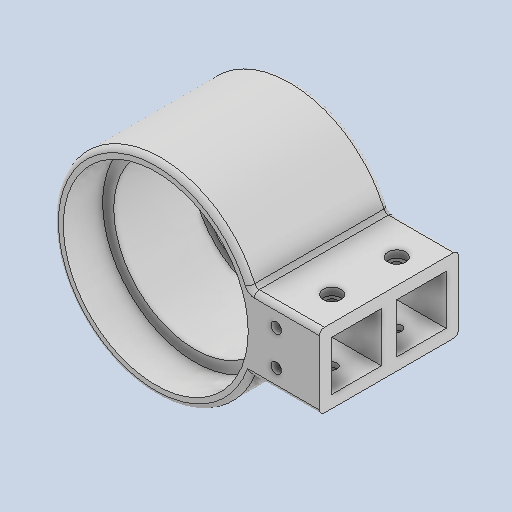
# Autodesk Inventor part: j2 arm part
Saved by Autodesk Inventor 2025 (Build 290162000, 162)
## iProperties
Created: 2025-07-06
Part Number: j2 arm part
Material: 一般
Document SubType Name: Modeling
Designer: gavin
Density: 1 g/cm^3
Appearance: 預設
Author: gavin
## iProperties of the stored document j2 arm part_3D 列印.ipt
Created: 2025-08-02
Part Number: j2 arm part_3D 列印
Material: 一般
Document SubType Name: Modeling
Designer: gavin
Density: 1 g/cm^3
Appearance: 預設
Author: gavin
Autodesk Inventor part; units mm, degrees
sketch "草圖1" plane through (0, 0, 0) normal (0, 0, 1) x (1, 0, 0)
  circle A0 centre (0, 0) radius 19.6
  circle A1 centre (0, 0) radius 41.575
  dimension "d0" = 39.2
  dimension "d1" = 83.15
  constraints: 2 centre point, 2 coincident
  measures "d0" diameter of A0
  measures "d1" diameter of A1
extrude "擠出1" add sketch "草圖1" along normal blind 5
sketch "草圖2" plane through (0, 0, 0) normal (0, 0, -1) x (-1, 0, 0)
  circle A0 centre (0, 0) radius 41.575 projected
extrude "擠出2" add sketch "草圖2" along normal blind 4
sketch "草圖4" plane through (0, 0, 5) normal (0, 0, 1) x (1, 0, 0)
  circle A0 centre (0, 0) radius 41.575 projected
  circle A1 centre (0, 0) radius 37.575
  dimension "d14" = 4
  constraints: 1 centre point
  measures "d14" radial gap between concentric circles of A0 A1
extrude "擠出4" add sketch "草圖4" along normal blind 47.5
sketch "草圖5" plane through (0, 0, 5) normal (0, 0, 1) x (1, 0, 0)
  circle A0 centre (0, 0) radius 37.575 projected
  circle A1 centre (0, 0) radius 33.075
  dimension "d17" = 4.5
  constraints: 1 centre point
  measures "d17" radial gap between concentric circles of A0 A1
extrude "擠出5" add sketch "草圖5" along normal blind 31.5
sketch "草圖6" plane through (0, 0, -4) normal (0, 0, -1) x (-1, 0, 0)
  line L0 (-66.575, 15.075) -> (-66.575, -15.075)
  line L1 (-66.575, 15.075) -> (-38.7456, 15.075)
  circle A0 centre (0, 0) radius 41.575 projected
  line L2 (-66.575, -15.075) -> (-38.7456, -15.075)
  point P0 (-41.575, 0)
  dimension "d20" = 30.15
  dimension "d22" = 15.075
  dimension "d25" = 25
  constraints: 6 end point, 3 point on circle, 2 horizontal, 1 vertical
  measures "d20" distance of L0.start L0.end
  measures "d22" distance from line of point (0, 0) L1
  measures "d25" distance from line of point (-41.575, 0) L0
extrude "擠出6" add sketch "草圖6" against normal up to surface (56.5 mm away) contours L1 A0 L2 L0
sketch "草圖7" plane through (66.575, -15.075, -4) normal (1, 0, 0) x (0, 0, -1)
  line L0 (-56.5, 30.15) -> (-56.5, 0) projected
  line L1 (0, 0) -> (-56.5, 0) projected
  line L2 (0, 30.15) -> (0, 0) projected
  line L3 (0, 30.15) -> (-56.5, 30.15) projected
  line L4 (-51.5, 5) -> (-31.35, 5)
  line L5 (-31.35, 5) -> (-31.35, 25.15)
  line L6 (-31.35, 25.15) -> (-51.5, 25.15)
  line L7 (-51.5, 25.15) -> (-51.5, 5)
  line L8 (-51.5, 5) -> (-31.35, 25.15) construction
  line L9 (-31.35, 5) -> (-51.5, 25.15) construction
  line L10 (-25.15, 5.0185) -> (-5, 5.0185)
  line L11 (-5, 5.0185) -> (-5, 25.15)
  line L12 (-5, 25.15) -> (-25.15, 25.15)
  line L13 (-25.15, 25.15) -> (-25.15, 5.0185)
  line L14 (-25.15, 5.0185) -> (-5, 25.15) construction
  line L15 (-5, 5.0185) -> (-25.15, 25.15) construction
  point P0 (-4, 15.075)
  point P1 (-41.425, 15.075)
  point P2 (-15.075, 15.0842)
  dimension "d26" = 20.15
  dimension "d27" = 20.15
  dimension "d28" = 20.15
  dimension "d29" = 5
  dimension "d30" = 5
  dimension "d31" = 5
  constraints: 24 end point, 4 midpoint, 4 parallel, 2 horizontal, 2 perpendicular, 1 point on line
  measures "d26" distance of L5.end L6.end
  measures "d27" distance of L6.end L4.start
  measures "d28" distance of L11.end L12.end
  measures "d29" distance between parallel lines of L0 L7
  measures "d30" distance between parallel lines of L6 L3
  measures "d31" distance between parallel lines of L2 L11
extrude "擠出7" cut sketch "草圖7" against normal blind 20 contours L7 L6 L5 L4 | L13 L12 L11 L10
fillet "圓角1" radius 2 7 edges at (52.6603, 15.075, -4) (-41.575, 0, -4) (52.6603, -15.075, -4) (38.7456, 15.075, 24.25) (52.6603, 15.075, 52.5) (-41.575, 0, 52.5) (52.6603, -15.075, 52.5)
sketch "草圖8" plane through (0, 0, 52.5) normal (0, 0, 1) x (1, 0, 0)
  line L0 (52.9465, -6.0747) -> (44.9865, -6.0635) projected
  line L1 (52.9465, -6.0747) -> (52.9551, 0.0253) projected
  line L2 (44.9951, 0.0365) -> (52.9551, 0.0253) projected
  line L3 (44.9865, -6.0635) -> (44.9951, 0.0365) projected
  circle A0 centre (48.975, -7.075) radius 2.165
  circle A1 centre (48.975, 7.075) radius 2.165
  line L4 (38.7456, -15.075) -> (66.575, -15.075) projected
  line L5 (66.575, 15.075) -> (40.0902, 15.075) projected
  point P0 (0, 0)
  dimension "d36" = 4.33
  dimension "d37" = 4.33
  dimension "d38" = 8
  dimension "d39" = 8
  constraints: 2 centre point
  measures "d36" diameter of A0
  measures "d37" diameter of A1
  measures "d38" distance from line of L4 A0.centre
  measures "d39" distance from line of L5 A1.centre
extrude "擠出8" cut sketch "草圖8" against normal up to surface (5 mm away) contours A0 L0 | L0 A0 | A1
sketch "草圖9" plane through (38.7456, -15.075, 50.5) normal (0, -1, 0) x (1, 0, 0)
  line L0 (27.8294, -29.35) -> (27.8294, -49.5) projected
  line L1 (27.8294, -29.35) -> (7.8294, -29.35) projected
  line L2 (7.8294, -29.35) -> (7.8294, -49.5) projected
  line L3 (27.8294, -49.5) -> (7.8294, -49.5) projected
  line L4 (27.8294, -3) -> (27.8294, -23.15) projected
  line L5 (27.8294, -3) -> (7.8294, -3) projected
  line L6 (7.8294, -3) -> (7.8294, -23.15) projected
  line L7 (27.8294, -23.15) -> (7.8294, -23.15) projected
  circle A0 centre (17.8294, -39.425) radius 2.1
  circle A1 centre (17.8294, -13.075) radius 2.1
  point P0 (-38.7456, -50.5)
  dimension "d42" = 4.2
  dimension "d43" = 4.2
  constraints: 2 centre point
  measures "d42" diameter of A0
  measures "d43" diameter of A1
extrude "擠出9" cut sketch "草圖9" against normal through all contours A0 | A1
sketch "草圖10" plane through (38.7456, -15.075, 50.5) normal (0, -1, 0) x (1, 0, 0)
  circle A0 centre (17.8294, -39.425) radius 2.1 projected
  circle A1 centre (17.8294, -39.425) radius 3.65
  circle A2 centre (17.8294, -13.075) radius 2.1 projected
  circle A3 centre (17.8294, -13.075) radius 3.65
  point P0 (-38.7456, -50.5)
  dimension "d46" = 7.3
  dimension "d47" = 7.3
  constraints: 2 centre point, 2 coincident
  measures "d46" diameter of A1
  measures "d47" diameter of A3
extrude "擠出10" cut sketch "草圖10" against normal blind 3
mirror "鏡射1" about plane through (0, 0, 0) normal (0, 1, 0) of "擠出10"
sketch "草圖14" plane through (0, 0, 5) normal (0, 0, 1) x (1, 0, 0)
  circle A0 centre (0, 0) radius 19.6 projected
extrude "擠出13" add sketch "草圖14" against normal up to surface (9 mm away)
sketch "草圖15" plane through (0, 0, -4) normal (0, 0, -1) x (-1, 0, 0)
  circle A0 centre (0, 0) radius 13.5
  dimension "d64" = 27
  constraints: 1 centre point, 1 coincident
  measures "d64" diameter of A0
extrude "擠出14" cut sketch "草圖15" against normal up to surface (9 mm away)
sketch "草圖16" plane through (0, 0, 5) normal (0, 0, 1) x (1, 0, 0)
  circle A0 centre (0, 0) radius 18.415
  circle A1 centre (0, 0) radius 13.5 projected
  constraints: 1 centre point
ref_plane "工作平面2" through (-13.4156, -13.4156, 7) normal (0, 0, 1) x (1, -0.0000484, 0)
extrude "擠出15" add sketch "草圖16" along normal up to surface (2 mm away)
ref_plane "工作平面3" through (0, 0, 7) normal (0, 0, 1) x (1, 0, 0)
sketch "草圖17" plane through (0, 0, 7) normal (0, 0, 1) x (1, 0, 0)
  circle A0 centre (0, 0) radius 7.575
  circle A1 centre (0, 0) radius 18.415 projected
  dimension "d71" = 15.15
  constraints: 1 centre point, 1 coincident
  measures "d71" diameter of A0
extrude "擠出16" add sketch "草圖17" along normal blind 3
sketch "草圖18" plane through (0, 0, 10) normal (0, 0, 1) x (1, 0, 0)
  circle A0 centre (0, 0) radius 7.575 projected
  circle A1 centre (0, 0) radius 10.575
  point P0 (0, 0)
  dimension "d74" = 3
  constraints: 1 centre point
  measures "d74" radial gap between concentric circles of A0 A1
ref_plane "工作平面4" through (-7.4754, -7.4754, 19) normal (0, 0, 1) x (1, -0.0000484, 0)
extrude "擠出17" add sketch "草圖18" along normal up to surface (9 mm away)
fillet "圓角3" radius 3 2 edges at (-18.415, 0, 5) (-10.575, 0, 10)
chamfer "倒角1" distance 1 angle 45 1 edges at (13.5, 0, -4)
equation "\"d22\" = 0.5 * d20"
equation "\"d27\" = d26"
equation "\"d28\" = d26"
